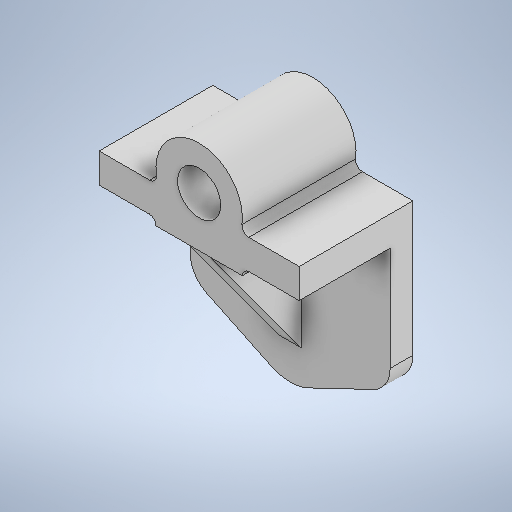
# Autodesk Inventor part: cad@50
Saved by Autodesk Inventor 2025.2 (Build 292293000, 293)
## iProperties
Created: 2025-04-09
Part Number: cad@50
Material: Generic
Document SubType Name: Modeling
Designer: spars
Density: 1 g/cm^3
Appearance: Default
Author: spars
Autodesk Inventor part; units mm, degrees
ref_plane "YZ Plane" through (0, 0, 0) normal (1, 0, 0) x (0, 1, 0)
ref_plane "XZ Plane" through (0, 0, 0) normal (0, 1, 0) x (-1, 0, 0)
sketch "Sketch1" plane through (0, 0, 0) normal (0, 0, 1) x (1, 0, 0)
  line L0 (-350.0309, 61.9823) -> (-142.1563, 61.9823) construction
  line L1 (-142.1563, 61.9823) -> (-142.1563, -104.6138) construction
  line L2 (-142.1563, -104.6138) -> (-350.0309, -104.6138) construction
  line L3 (-350.0309, -104.6138) -> (-350.0309, 61.9823) construction
  line L4 (-44, 33.5) -> (44, 33.5)
  line L5 (44, 33.5) -> (44, -25.3108)
  line L6 (-44, -25.3108) -> (-44, 33.5)
  line L7 (-44, 33.5) -> (44, -33.5) construction
  line L8 (44, 33.5) -> (-44, -33.5) construction
  arc A0 (-8.2045, -50.6373) -> (8.2045, -50.6373) centre (0, -33.5) ccw
  line L9 (-36.6136, -37.0363) -> (-8.2045, -50.6373)
  line L10 (36.6136, -37.0363) -> (8.2045, -50.6373)
  arc A1 (-44, -25.3108) -> (-36.6136, -37.0363) centre (-31, -25.3108) ccw
  arc A2 (36.6136, -37.0363) -> (44, -25.3108) centre (31, -25.3108) ccw
  point P0 (0, 0)
  dimension "d5" = 88
  dimension "d6" = 67
  dimension "d7" = 38
  dimension "d9" = 13
  constraints: 14 end point, 6 point on circle, 6 tangent, 4 point on line, 3 centre point, 2 midpoint, 1 equal radius, 1 horizontal, 1 parallel, 1 perpendicular, 2 other
  measures "d5" distance of L7.end L8.end
  measures "d6" distance of L4.end L7.end
  measures "d7" diameter of A0
  measures "d9" radius of A1
extrude "Extrusion1" add sketch "Sketch1" along normal blind 10
sketch "Sketch2" plane through (0, 0, 10) normal (0, 0, 1) x (1, 0, 0)
  line L0 (44, 33.5) -> (-44, 33.5) projected
  line L1 (44, -25.3108) -> (44, 33.5) projected
  line L2 (-44, 33.5) -> (44, 33.5)
  line L3 (44, 33.5) -> (44, 20.5)
  line L4 (44, 20.5) -> (-44, 20.5)
  line L5 (-44, 20.5) -> (-44, 33.5)
  point P0 (0, 0)
  dimension "d12" = 13
  constraints: 8 end point, 2 parallel, 1 horizontal, 1 perpendicular, 1 point on line
  measures "d12" distance of L2.end L3.end
extrude "Extrusion2" add sketch "Sketch2" along normal blind 40
sketch "Sketch3" plane through (-44, 20.5, 10) normal (0, -1, 0) x (1, 0, 0)
  point P0 (44, -10)
ref_plane "Work Plane1" through (0, -25.3108, 0) normal (1, 0, 0) x (0, 0, -1)
sketch "Sketch4" plane through (0, -25.3108, 0) normal (1, 0, 0) x (0, 0, -1)
  line L0 (-10, 45.8108) -> (-50, 45.8108) projected
  line L1 (-10, -25.3265) -> (-10, -27.1892) projected
  line L2 (-50, 45.8108) -> (-50, 58.8108) projected
  line L3 (-10, -25.3265) -> (-10, -11.7255) projected
  line L4 (-50, 42.8108) -> (-50, 44.8157)
  line L5 (-50, 42.8108) -> (-42.3694, 32.4072)
  point P0 (0, 25.3108)
  dimension "d43" = 3
  constraints: 4 end point, 1 vertical
  measures "d43" distance of L0.end L4.start
extrude "Rib1" add sketch "Sketch4" along normal mid plane 10 rib yes fills toward (-49.95, 43.8133) open curves L4 L5
sketch "Sketch5" plane through (-44, 20.5, 10) normal (0, -1, 0) x (1, 0, 0)
  line L0 (39, 0) -> (39, 40) projected
  line L1 (39, 0) -> (0, 0) projected
  line L2 (39, 40) -> (25, 40)
  line L3 (25, 40) -> (25, 0)
  line L4 (25, 0) -> (39, 0)
  line L5 (39, 0) -> (39, 40)
  line L6 (49, 0) -> (49, 40) projected
  line L7 (49, 40) -> (63, 40)
  line L8 (63, 40) -> (63, 0)
  line L9 (63, 0) -> (49, 0)
  line L10 (49, 0) -> (49, 40)
  point P0 (44, -10)
  dimension "d21" = 14
  dimension "d22" = 14
  constraints: 16 end point, 4 parallel, 2 horizontal, 2 perpendicular, 2 point on line
  measures "d21" distance of L4.end L3.end
  measures "d22" distance of L8.end L9.end
extrude "Extrusion3" add sketch "Sketch5" along normal blind 3
fillet "Face Fillet1" radius 3 1 edges at (-19, 20.5, 30)
fillet "Face Fillet2" radius 3 1 edges at (19, 20.5, 30)
ref_plane "Work Plane2" through (0, 0, 50) normal (0, 0, 1) x (1, 0, 0)
sketch "Sketch6" plane through (0, 0, 50) normal (0, 0, 1) x (1, 0, 0)
  line L0 (-411.8636, 122.6575) -> (-209.6493, 122.6575) construction
  line L1 (-209.6493, 122.6575) -> (-209.6493, -39.4022) construction
  line L2 (-209.6493, -39.4022) -> (-411.8636, -39.4022) construction
  line L3 (-411.8636, -39.4022) -> (-411.8636, 122.6575) construction
  circle A0 centre (0, 39.5) radius 9.5
  arc A1 (18.8225, 36.9091) -> (-18.8225, 36.9091) centre (0, 39.5) ccw
  line L4 (44, 33.5) -> (-44, 33.5) projected
  line L5 (22, 20.5) -> (44, 20.5) projected
  line L6 (-44, 33.5) -> (-44, 20.5) projected
  line L7 (21.7945, 33.5) -> (44, 33.5)
  arc A2 (-21.7945, 33.5) -> (-18.8225, 36.9091) centre (-21.7945, 36.5) ccw
  arc A3 (18.8225, 36.9091) -> (21.7945, 33.5) centre (21.7945, 36.5) ccw
  line L8 (-21.7945, 33.5) -> (-7.3655, 33.5)
  line L9 (7.3655, 33.5) -> (21.7945, 33.5)
  point P0 (0, 0)
  point P1 (33, 20.5)
  point P2 (-18.0278, 33.5)
  point P3 (18.0278, 33.5)
  dimension "d33" = 19
  dimension "d34" = 38
  dimension "d36" = 19
  dimension "d37" = 3
  constraints: 10 point on circle, 6 end point, 4 centre point, 4 tangent, 3 point on line, 2 collinear, 1 coincident, 1 equal radius, 1 midpoint, 2 other
  measures "d33" diameter of A0
  measures "d34" diameter of A1
  measures "d36" vertical distance of point (33, 20.5) A0.centre
  measures "d37" radius of A2
extrude "Extrusion4" add sketch "Sketch6" against normal blind 50 contours A0 L4 A2 A1 A3
sketch "Sketch7" plane through (0, 0, 50) normal (0, 0, 1) x (1, 0, 0)
  arc A0 (7.3655, 33.5) -> (-7.3655, 33.5) centre (0, 39.5) ccw projected
  circle A1 centre (0, 39.5) radius 9.5
  point P0 (0, 0)
  point P1 (-7.3655, 33.5)
  dimension "d40" = 19
  constraints: 1 centre point, 1 coincident
  measures "d40" diameter of A1
extrude "Extrusion5" cut sketch "Sketch7" against normal blind 50
body "Solid1"
